Autodesk Fusion 360 part; units mm, degrees
(part 2 of 4)
sketch "Esboço4" plane through (0, 0, 2) normal (0, 0, 1) x (-1, 0, 0)
  arc A0 (-38.7303, -7.6383) -> (-38.142, -9.266) centre (-36.7404, -7.8393) ccw
  arc A1 (-38.7303, -7.6383) -> (-38.7376, 7.7103) centre (-114.3455, 0) ccw
  arc A2 (-38.1438, 9.3455) -> (-38.7376, 7.7103) centre (-36.7479, 7.9132) ccw
  line L0 (-38.1438, 9.3455) -> (-27.9241, 19.3052)
  arc A3 (-24.5283, 17.871) -> (-27.9241, 19.3052) centre (-26.5283, 17.8728) ccw
  line L1 (-24.5283, 17.871) -> (-24.5606, -17.8415)
  arc A4 (-27.9622, -19.2664) -> (-24.5607, -17.8415) centre (-26.5606, -17.8397) ccw
  line L2 (-27.9622, -19.2664) -> (-38.142, -9.266)
  line L3 (19.3052, -27.9241) -> (9.3455, -38.1438)
  arc A5 (7.7103, -38.7376) -> (9.3455, -38.1438) centre (7.9132, -36.7479) ccw
  arc A6 (7.7103, -38.7376) -> (-7.6383, -38.7303) centre (0, -114.3455) ccw
  arc A7 (-9.266, -38.142) -> (-7.6383, -38.7303) centre (-7.8393, -36.7404) ccw
  line L4 (-9.266, -38.142) -> (-19.2664, -27.9622)
  arc A8 (-17.8415, -24.5606) -> (-19.2664, -27.9622) centre (-17.8397, -26.5606) ccw
  line L5 (-17.8415, -24.5606) -> (17.871, -24.5283)
  arc A9 (19.3052, -27.9241) -> (17.871, -24.5283) centre (17.8728, -26.5283) ccw
  arc A10 (37.4337, 15.5639) -> (40.6601, 16.1647) centre (38.8376, 16.9884) ccw
  line L6 (37.4337, 15.5639) -> (14.6425, 38.0264)
  arc A11 (15.1963, 41.2612) -> (14.6425, 38.0264) centre (16.0464, 39.4508) ccw
  line L7 (15.1963, 41.2612) -> (28.3187, 47.4234)
  arc A12 (34.7856, 45.3775) -> (28.3187, 47.4234) centre (30.444, 42.8975) ccw
  arc A13 (34.7856, 45.3775) -> (44.4886, 35.8486) centre (56.4937, 57.7776) ccw
  arc A14 (46.6438, 29.4035) -> (44.4886, 35.8486) centre (42.0875, 31.4628) ccw
  line L8 (46.6438, 29.4035) -> (40.6601, 16.1647)
  line L9 (41.7895, -17.0192) -> (61.9965, -63.6935)
  arc A15 (55.3948, -68.0303) -> (61.9965, -63.6935) centre (58.3475, -65.3318) ccw
  line L10 (55.3948, -68.0303) -> (23.5953, -33.2362)
  arc A16 (23.7067, -29.0729) -> (23.5953, -33.2362) centre (25.8097, -31.2123) ccw
  line L11 (23.7067, -29.0729) -> (36.9334, -16.0716)
  arc A17 (41.7895, -17.0192) -> (36.9334, -16.0716) centre (39.0364, -18.2111) ccw
  arc A18 (9.266, 38.142) -> (7.6383, 38.7303) centre (7.8393, 36.7404) ccw
  line L12 (9.266, 38.142) -> (19.2664, 27.9622)
  arc A19 (17.8415, 24.5606) -> (19.2664, 27.9622) centre (17.8397, 26.5606) ccw
  line L13 (17.8415, 24.5606) -> (-17.871, 24.5283)
  arc A20 (-19.3052, 27.9241) -> (-17.871, 24.5283) centre (-17.8728, 26.5283) ccw
  line L14 (-19.3052, 27.9241) -> (-9.3455, 38.1438)
  arc A21 (-7.7103, 38.7376) -> (-9.3455, 38.1438) centre (-7.9132, 36.7479) ccw
  arc A22 (-7.7103, 38.7376) -> (7.6383, 38.7303) centre (0, 114.3455) ccw
  arc A23 (38.1376, -9.2791) -> (38.7256, -7.6527) centre (36.7356, -7.8528) ccw
  line L15 (38.1376, -9.2791) -> (27.9736, -19.2699)
  arc A24 (24.5716, -17.8424) -> (27.9736, -19.2699) centre (26.5716, -17.8436) ccw
  line L16 (24.5716, -17.8424) -> (24.5916, 17.8264)
  arc A25 (27.9955, 19.2498) -> (24.5916, 17.8264) centre (26.5916, 17.8253) ccw
  line L17 (27.9955, 19.2498) -> (38.1463, 9.2454)
  arc A26 (38.7321, 7.6192) -> (38.1463, 9.2454) centre (36.7424, 7.821) ccw
  arc A27 (38.7321, 7.6192) -> (38.7256, -7.6527) centre (114.3432, -0.0492) ccw
  arc A28 (-61.9967, -63.6938) -> (-55.4143, -68.0759) centre (-58.3695, -65.3802) ccw
  line L18 (-61.9967, -63.6938) -> (-41.8922, -17.2564)
  arc A29 (-36.246, -16.5772) -> (-41.8922, -17.2564) centre (-38.8636, -18.6251) ccw
  line L19 (-36.246, -16.5772) -> (-23.6374, -29.1331)
  arc A30 (-23.5625, -33.2372) -> (-23.6374, -29.1331) centre (-25.7596, -31.2246) ccw
  line L20 (-23.5625, -33.2372) -> (-55.4143, -68.0759)
  line L21 (5, -97.464) -> (5, -58.6595)
  arc A31 (7, -56.6595) -> (5, -58.6595) centre (7, -58.6595) ccw
  line L22 (7, -56.6595) -> (10.473, -56.6595)
  arc A32 (14.3032, -58.4456) -> (10.473, -56.6595) centre (10.473, -61.6595) ccw
  line L23 (14.3032, -58.4456) -> (34.3305, -82.3132)
  arc A33 (35.4243, -86.3954) -> (34.3305, -82.3132) centre (30.5003, -85.5271) ccw
  line L24 (35.4243, -86.3954) -> (32.7648, -101.4781)
  arc A34 (26.9725, -105.5339) -> (32.7648, -101.4781) centre (27.8408, -100.6098) ccw
  line L25 (26.9725, -105.5339) -> (9.1318, -102.3881)
  arc A35 (5, -97.464) -> (9.1318, -102.3881) centre (10, -97.464) ccw
  arc A36 (-40.9054, 16.7074) -> (-37.3489, 15.6517) centre (-38.8619, 17.0732) ccw
  line L26 (-40.9054, 16.7074) -> (-46.7322, 29.5993)
  arc A37 (-44.339, 36.0244) -> (-46.7322, 29.5993) centre (-42.0339, 31.5075) ccw
  arc A38 (-44.339, 36.0244) -> (-34.6129, 45.4956) centre (-56.2565, 57.9923) ccw
  arc A39 (-28.1234, 47.5076) -> (-34.6129, 45.4956) centre (-30.28, 42.9921) ccw
  line L27 (-28.1234, 47.5076) -> (-14.9942, 41.2515)
  arc A40 (-14.46, 38.0146) -> (-14.9942, 41.2515) centre (-15.8549, 39.4469) ccw
  line L28 (-14.46, 38.0146) -> (-37.3489, 15.6517)
  line L29 (70.4711, -73.2) -> (50.5773, -27.2494)
  arc A41 (51.0282, 29.3922) -> (50.5773, -27.2494) centre (114.8154, 0.5617) ccw
  line L30 (51.0282, 29.3922) -> (70.7852, 73.1043)
  arc A42 (70.7852, 73.1043) -> (60.1979, 89.9288) centre (75, 87.5) ccw
  arc A43 (35.9657, 79.8952) -> (60.1979, 89.9288) centre (-0.31, 201.7835) ccw
  arc A44 (-60.2098, 89.9999) -> (-70.7852, 73.1043) centre (-75, 87.5) ccw
  line L31 (-70.7852, 73.1043) -> (-51.0282, 29.3922)
  arc A45 (-50.5773, -27.2494) -> (-51.0282, 29.3922) centre (-114.8154, 0.5617) ccw
  line L32 (-50.5773, -27.2494) -> (-70.4711, -73.2)
  arc A46 (-70.4711, -73.2) -> (-73.7447, -102.4474) centre (-75, -87.5) ccw
  arc A47 (-46.7294, -108.889) -> (-73.7447, -102.4474) centre (-70.0264, -146.7235) ccw
  arc A48 (72.6915, -102.3213) -> (44.7852, -108.3244) centre (66.5604, -141.6847) ccw
  arc A49 (72.6915, -102.3213) -> (70.4711, -73.2) centre (75, -87.5) ccw
  arc A50 (-10.473, -56.6595) -> (-14.3032, -58.4456) centre (-10.473, -61.6595) ccw
  line L33 (-10.473, -56.6595) -> (-7, -56.6595)
  arc A51 (-5, -58.6595) -> (-7, -56.6595) centre (-7, -58.6595) ccw
  line L34 (-5, -58.6595) -> (-5, -97.464)
  arc A52 (-9.1318, -102.3881) -> (-5, -97.464) centre (-10, -97.464) ccw
  line L35 (-9.1318, -102.3881) -> (-26.9725, -105.5339)
  arc A53 (-32.7648, -101.4781) -> (-26.9725, -105.5339) centre (-27.8408, -100.6098) ccw
  line L36 (-32.7648, -101.4781) -> (-35.4243, -86.3954)
  arc A54 (-34.3305, -82.3132) -> (-35.4243, -86.3954) centre (-30.5003, -85.5271) ccw
  line L37 (-34.3305, -82.3132) -> (-14.3032, -58.4456)
  circle A55 centre (-40.65, 60) radius 2.15
  line L38 (47.15, 42.4858) -> (47.15, 67.561)
  arc A56 (49.4611, 71.7764) -> (47.15, 67.561) centre (52.15, 67.561) ccw
  line L39 (49.4611, 71.7764) -> (57.5607, 76.943)
  arc A57 (64.8173, 70.6939) -> (57.5607, 76.943) centre (60.2496, 72.7276) ccw
  line L40 (64.8173, 70.6939) -> (51.1653, 40.0309)
  arc A58 (49.5538, 39.7214) -> (51.1653, 40.0309) centre (50.2517, 40.4376) ccw
  line L41 (49.5538, 39.7214) -> (47.4521, 41.7697)
  arc A59 (47.15, 42.4858) -> (47.4521, 41.7697) centre (48.15, 42.4858) ccw
  circle A60 centre (40.65, 60) radius 2.15
  circle A61 centre (-40.65, 50) radius 2.15
  arc A62 (-57.5607, 76.943) -> (-64.8173, 70.6939) centre (-60.2496, 72.7276) ccw
  line L42 (-57.5607, 76.943) -> (-49.4611, 71.7764)
  arc A63 (-47.15, 67.561) -> (-49.4611, 71.7764) centre (-52.15, 67.561) ccw
  line L43 (-47.15, 67.561) -> (-47.15, 42.4858)
  arc A64 (-47.4521, 41.7697) -> (-47.15, 42.4858) centre (-48.15, 42.4858) ccw
  line L44 (-47.4521, 41.7697) -> (-49.5538, 39.7214)
  arc A65 (-51.1653, 40.0309) -> (-49.5538, 39.7214) centre (-50.2517, 40.4376) ccw
  line L45 (-51.1653, 40.0309) -> (-64.8173, 70.6939)
  circle A66 centre (40.65, 50) radius 2.15
  line L46 (8, -50.7) -> (-8, -42.5) construction
  line L47 (0, -46.6) -> (-20, -46.6) construction
  arc A67 (-9.266, -38.142) -> (-7.6383, -38.7303) centre (-7.8393, -36.7404) ccw
  line L48 (-8, -50.7) -> (-8, -42.5)
  line L49 (-8, -42.5) -> (8, -42.5)
  circle A68 centre (-10.25, -46.6) radius 1.5
  line L50 (8, -50.7) -> (-8, -50.7)
  line L51 (0, -46.6) -> (20, -46.6) construction
  arc A69 (7.7103, -38.7376) -> (9.3455, -38.1438) centre (7.9132, -36.7479) ccw
  line L52 (-8, -50.7) -> (8, -42.5) construction
  arc A70 (7.7103, -38.7376) -> (-7.6383, -38.7303) centre (0, -114.3455) ccw
  line L53 (8, -42.5) -> (8, -50.7)
  circle A71 centre (10.25, -46.6) radius 1.5
  line L54 (8.1464, -6.7322) -> (2.1213, -0.7071)
  arc A72 (2.1213, 0.7071) -> (2.1213, -0.7071) centre (2.8284, 0) ccw
  line L55 (2.1213, 0.7071) -> (8.1464, 6.7322)
  arc A73 (9, 6.3787) -> (8.1464, 6.7322) centre (8.5, 6.3787) ccw
  line L56 (9, 6.3787) -> (9, -6.3787)
  arc A74 (8.1464, -6.7322) -> (9, -6.3787) centre (8.5, -6.3787) ccw
  arc A75 (-6.7322, -8.1464) -> (-6.3787, -9) centre (-6.3787, -8.5) ccw
  line L57 (-6.7322, -8.1464) -> (-0.7071, -2.1213)
  arc A76 (0.7071, -2.1213) -> (-0.7071, -2.1213) centre (0, -2.8284) ccw
  line L58 (0.7071, -2.1213) -> (6.7322, -8.1464)
  arc A77 (6.3787, -9) -> (6.7322, -8.1464) centre (6.3787, -8.5) ccw
  line L59 (6.3787, -9) -> (-6.3787, -9)
  arc A78 (-8.1464, 6.7322) -> (-9, 6.3787) centre (-8.5, 6.3787) ccw
  line L60 (-8.1464, 6.7322) -> (-2.1213, 0.7071)
  arc A79 (-2.1213, -0.7071) -> (-2.1213, 0.7071) centre (-2.8284, 0) ccw
  line L61 (-2.1213, -0.7071) -> (-8.1464, -6.7322)
  arc A80 (-9, -6.3787) -> (-8.1464, -6.7322) centre (-8.5, -6.3787) ccw
  line L62 (-9, -6.3787) -> (-9, 6.3787)
  arc A81 (6.7322, 8.1464) -> (6.3787, 9) centre (6.3787, 8.5) ccw
  line L63 (6.7322, 8.1464) -> (0.7071, 2.1213)
  arc A82 (-0.7071, 2.1213) -> (0.7071, 2.1213) centre (0, 2.8284) ccw
  line L64 (-0.7071, 2.1213) -> (-6.7322, 8.1464)
  arc A83 (-6.3787, 9) -> (-6.7322, 8.1464) centre (-6.3787, 8.5) ccw
  line L65 (-6.3787, 9) -> (6.3787, 9)
  line L66 (35.9657, 79.8952) -> (2.1827, 93.0889)
  arc A84 (2.1827, 93.0889) -> (-2.1423, 93.1045) centre (0, 87.5) ccw
  line L67 (0, 81.5) -> (15.6612, 75.3836)
  line L68 (-16.4256, 75.2214) -> (0, 81.5)
  line L69 (-2.1423, 93.1045) -> (-36.9275, 79.8081)
  arc A85 (-60.2098, 89.9999) -> (-36.7745, 80.3179) centre (-0.31, 201.7835) ccw
  circle A86 centre (0, 87.5) radius 2.15
  arc A87 (26.2105, 50.915) -> (27.5676, 55.0697) centre (24.9353, 53.6305) ccw
  line L70 (26.2105, 50.915) -> (10.6059, 43.5872)
  arc A88 (9.3307, 43.3027) -> (10.6059, 43.5872) centre (9.3307, 46.3027) ccw
  line L71 (9.3307, 43.3027) -> (-9.3218, 43.3027)
  arc A89 (-10.6123, 43.5944) -> (-9.3218, 43.3027) centre (-9.3218, 46.3027) ccw
  line L72 (-10.6123, 43.5944) -> (-26.8632, 51.3381)
  arc A90 (-28.1945, 55.5044) -> (-26.8632, 51.3381) centre (-25.5727, 54.0463) ccw
  line L73 (-28.1945, 55.5044) -> (-17.9762, 73.8773)
  arc A91 (-16.4256, 75.2214) -> (-17.9762, 73.8773) centre (-15.3544, 72.4192) ccw
  arc A92 (17.2021, 74.0283) -> (15.6612, 75.3836) centre (14.5698, 72.5892) ccw
  line L74 (17.2021, 74.0283) -> (27.5676, 55.0697)
  arc A93 (-46.7294, -108.889) -> (-25.7561, -114.8285) centre (-25.7561, -74.8285) ccw
  line L75 (-25.7561, -114.8285) -> (22.9214, -114.8285)
  arc A94 (22.9214, -114.8285) -> (44.7852, -108.3244) centre (22.9214, -74.8285) ccw
  circle A95 centre (10, 10) radius 3
  circle A96 centre (-10, -10) radius 3
  circle A97 centre (10, -10) radius 3
  circle A98 centre (-10, 10) radius 3
  point P0 (0, -46.6)
  point P1 (0.156, 201.9423)
  point P2 (0.156, 201.9423)
  point P3 (0.156, 201.9423)
  point P4 (0.2929, 201.9885)
  point P5 (0.2929, 201.9885)
  point P6 (0.2929, 201.9885)
  point P7 (2.2046, 200.8918)
  point P8 (2.2046, 200.8918)
  dimension "d91" = 16
  dimension "d92" = 8.2
  dimension "d93" = 3
  dimension "d94" = 2.25
  dimension "d96" = 42.5
  dimension "d97" = 2.25
  constraint horizontal L50
  constraint perpendicular L48 L50
  constraint parallel L49 L50
  constraint parallel L48 L53
  constraint coincident P0 L46
  constraint coincident P0 L52
  constraint coincident P0 L47.start
  constraint perpendicular L47 L48
  constraint perpendicular L51 L53
  constraint coincident A71.centre L51
  measures "d91" distance of L46.end L49.end
  measures "d92" distance of L46.end L48.start
  measures "d93" diameter of A71
  measures "d94" distance of A71.centre L53
  measures "d96" distance of origin L49
  measures "d97" distance of A68.centre L48
extrude "Extrusão4" cut sketch "Esboço4" against normal through all contours L48 L49 L50 L53 | A68 | A71
sketch "Esboço5" plane through (0, 0, 2) normal (0, 0, 1) x (-1, 0, 0)
  circle A0 centre (40.65, 50) radius 2.15
  arc A1 (-57.5607, 76.943) -> (-64.8173, 70.6939) centre (-60.2496, 72.7276) ccw
  line L0 (-57.5607, 76.943) -> (-49.4611, 71.7764)
  arc A2 (-47.15, 67.561) -> (-49.4611, 71.7764) centre (-52.15, 67.561) ccw
  line L1 (-47.15, 67.561) -> (-47.15, 42.4858)
  arc A3 (-47.4521, 41.7697) -> (-47.15, 42.4858) centre (-48.15, 42.4858) ccw
  line L2 (-47.4521, 41.7697) -> (-49.5538, 39.7214)
  arc A4 (-51.1653, 40.0309) -> (-49.5538, 39.7214) centre (-50.2517, 40.4376) ccw
  line L3 (-51.1653, 40.0309) -> (-64.8173, 70.6939)
  circle A5 centre (-40.65, 50) radius 2.15
  circle A6 centre (40.65, 60) radius 2.15
  line L4 (47.15, 42.4858) -> (47.15, 67.561)
  arc A7 (49.4611, 71.7764) -> (47.15, 67.561) centre (52.15, 67.561) ccw
  line L5 (49.4611, 71.7764) -> (57.5607, 76.943)
  arc A8 (64.8173, 70.6939) -> (57.5607, 76.943) centre (60.2496, 72.7276) ccw
  line L6 (64.8173, 70.6939) -> (51.1653, 40.0309)
  arc A9 (49.5538, 39.7214) -> (51.1653, 40.0309) centre (50.2517, 40.4376) ccw
  line L7 (49.5538, 39.7214) -> (47.4521, 41.7697)
  arc A10 (47.15, 42.4858) -> (47.4521, 41.7697) centre (48.15, 42.4858) ccw
  circle A11 centre (-40.65, 60) radius 2.15
  arc A12 (-10.473, -56.6595) -> (-14.3032, -58.4456) centre (-10.473, -61.6595) ccw
  line L8 (-10.473, -56.6595) -> (-7, -56.6595)
  arc A13 (-5, -58.6595) -> (-7, -56.6595) centre (-7, -58.6595) ccw
  line L9 (-5, -58.6595) -> (-5, -97.464)
  arc A14 (-9.1318, -102.3881) -> (-5, -97.464) centre (-10, -97.464) ccw
  line L10 (-9.1318, -102.3881) -> (-26.9725, -105.5339)
  arc A15 (-32.7648, -101.4781) -> (-26.9725, -105.5339) centre (-27.8408, -100.6098) ccw
  line L11 (-32.7648, -101.4781) -> (-35.4243, -86.3954)
  arc A16 (-34.3305, -82.3132) -> (-35.4243, -86.3954) centre (-30.5003, -85.5271) ccw
  line L12 (-34.3305, -82.3132) -> (-14.3032, -58.4456)
  line L13 (70.4711, -73.2) -> (50.5773, -27.2494)
  arc A17 (51.0282, 29.3922) -> (50.5773, -27.2494) centre (114.8154, 0.5617) ccw
  line L14 (51.0282, 29.3922) -> (70.7852, 73.1043)
  arc A18 (70.7852, 73.1043) -> (60.1979, 89.9288) centre (75, 87.5) ccw
  arc A19 (35.9657, 79.8952) -> (60.1979, 89.9288) centre (-0.31, 201.7835) ccw
  arc A20 (-60.2098, 89.9999) -> (-70.7852, 73.1043) centre (-75, 87.5) ccw
  line L15 (-70.7852, 73.1043) -> (-51.0282, 29.3922)
  arc A21 (-50.5773, -27.2494) -> (-51.0282, 29.3922) centre (-114.8154, 0.5617) ccw
  line L16 (-50.5773, -27.2494) -> (-70.4711, -73.2)
  arc A22 (-70.4711, -73.2) -> (-73.7447, -102.4474) centre (-75, -87.5) ccw
  arc A23 (-46.7294, -108.889) -> (-73.7447, -102.4474) centre (-70.0264, -146.7235) ccw
  arc A24 (72.6915, -102.3213) -> (44.7852, -108.3244) centre (66.5604, -141.6847) ccw
  arc A25 (72.6915, -102.3213) -> (70.4711, -73.2) centre (75, -87.5) ccw
  arc A26 (-40.9054, 16.7074) -> (-37.3489, 15.6517) centre (-38.8619, 17.0732) ccw
  line L17 (-40.9054, 16.7074) -> (-46.7322, 29.5993)
  arc A27 (-44.339, 36.0244) -> (-46.7322, 29.5993) centre (-42.0339, 31.5075) ccw
  arc A28 (-44.339, 36.0244) -> (-34.6129, 45.4956) centre (-56.2565, 57.9923) ccw
  arc A29 (-28.1234, 47.5076) -> (-34.6129, 45.4956) centre (-30.28, 42.9921) ccw
  line L18 (-28.1234, 47.5076) -> (-14.9942, 41.2515)
  arc A30 (-14.46, 38.0146) -> (-14.9942, 41.2515) centre (-15.8549, 39.4469) ccw
  line L19 (-14.46, 38.0146) -> (-37.3489, 15.6517)
  line L20 (5, -97.464) -> (5, -58.6595)
  arc A31 (7, -56.6595) -> (5, -58.6595) centre (7, -58.6595) ccw
  line L21 (7, -56.6595) -> (10.473, -56.6595)
  arc A32 (14.3032, -58.4456) -> (10.473, -56.6595) centre (10.473, -61.6595) ccw
  line L22 (14.3032, -58.4456) -> (34.3305, -82.3132)
  arc A33 (35.4243, -86.3954) -> (34.3305, -82.3132) centre (30.5003, -85.5271) ccw
  line L23 (35.4243, -86.3954) -> (32.7648, -101.4781)
  arc A34 (26.9725, -105.5339) -> (32.7648, -101.4781) centre (27.8408, -100.6098) ccw
  line L24 (26.9725, -105.5339) -> (9.1318, -102.3881)
  arc A35 (5, -97.464) -> (9.1318, -102.3881) centre (10, -97.464) ccw
  arc A36 (-61.9967, -63.6938) -> (-55.4143, -68.0759) centre (-58.3695, -65.3802) ccw
  line L25 (-61.9967, -63.6938) -> (-41.8922, -17.2564)
  arc A37 (-36.246, -16.5772) -> (-41.8922, -17.2564) centre (-38.8636, -18.6251) ccw
  line L26 (-36.246, -16.5772) -> (-23.6374, -29.1331)
  arc A38 (-23.5625, -33.2372) -> (-23.6374, -29.1331) centre (-25.7596, -31.2246) ccw
  line L27 (-23.5625, -33.2372) -> (-55.4143, -68.0759)
  arc A39 (38.1376, -9.2791) -> (38.7256, -7.6527) centre (36.7356, -7.8528) ccw
  line L28 (38.1376, -9.2791) -> (27.9736, -19.2699)
  arc A40 (24.5716, -17.8424) -> (27.9736, -19.2699) centre (26.5716, -17.8436) ccw
  line L29 (24.5716, -17.8424) -> (24.5916, 17.8264)
  arc A41 (27.9955, 19.2498) -> (24.5916, 17.8264) centre (26.5916, 17.8253) ccw
  line L30 (27.9955, 19.2498) -> (38.1463, 9.2454)
  arc A42 (38.7321, 7.6192) -> (38.1463, 9.2454) centre (36.7424, 7.821) ccw
  arc A43 (38.7321, 7.6192) -> (38.7256, -7.6527) centre (114.3432, -0.0492) ccw
  arc A44 (9.266, 38.142) -> (7.6383, 38.7303) centre (7.8393, 36.7404) ccw
  line L31 (9.266, 38.142) -> (19.2664, 27.9622)
  arc A45 (17.8415, 24.5606) -> (19.2664, 27.9622) centre (17.8397, 26.5606) ccw
  line L32 (17.8415, 24.5606) -> (-17.871, 24.5283)
  arc A46 (-19.3052, 27.9241) -> (-17.871, 24.5283) centre (-17.8728, 26.5283) ccw
  line L33 (-19.3052, 27.9241) -> (-9.3455, 38.1438)
  arc A47 (-7.7103, 38.7376) -> (-9.3455, 38.1438) centre (-7.9132, 36.7479) ccw
  arc A48 (-7.7103, 38.7376) -> (7.6383, 38.7303) centre (0, 114.3455) ccw
  line L34 (41.7895, -17.0192) -> (61.9965, -63.6935)
  arc A49 (55.3948, -68.0303) -> (61.9965, -63.6935) centre (58.3475, -65.3318) ccw
  line L35 (55.3948, -68.0303) -> (23.5953, -33.2362)
  arc A50 (23.7067, -29.0729) -> (23.5953, -33.2362) centre (25.8097, -31.2123) ccw
  line L36 (23.7067, -29.0729) -> (36.9334, -16.0716)
  arc A51 (41.7895, -17.0192) -> (36.9334, -16.0716) centre (39.0364, -18.2111) ccw
  arc A52 (37.4337, 15.5639) -> (40.6601, 16.1647) centre (38.8376, 16.9884) ccw
  line L37 (37.4337, 15.5639) -> (14.6425, 38.0264)
  arc A53 (15.1963, 41.2612) -> (14.6425, 38.0264) centre (16.0464, 39.4508) ccw
  line L38 (15.1963, 41.2612) -> (28.3187, 47.4234)
  arc A54 (34.7856, 45.3775) -> (28.3187, 47.4234) centre (30.444, 42.8975) ccw
  arc A55 (34.7856, 45.3775) -> (44.4886, 35.8486) centre (56.4937, 57.7776) ccw
  arc A56 (46.6438, 29.4035) -> (44.4886, 35.8486) centre (42.0875, 31.4628) ccw
  line L39 (46.6438, 29.4035) -> (40.6601, 16.1647)
  line L40 (19.3052, -27.9241) -> (9.3455, -38.1438)
  arc A57 (7.7103, -38.7376) -> (9.3455, -38.1438) centre (7.9132, -36.7479) ccw
  arc A58 (7.7103, -38.7376) -> (-7.6383, -38.7303) centre (0, -114.3455) ccw
  arc A59 (-9.266, -38.142) -> (-7.6383, -38.7303) centre (-7.8393, -36.7404) ccw
  line L41 (-9.266, -38.142) -> (-19.2664, -27.9622)
  arc A60 (-17.8415, -24.5606) -> (-19.2664, -27.9622) centre (-17.8397, -26.5606) ccw
  line L42 (-17.8415, -24.5606) -> (17.871, -24.5283)
  arc A61 (19.3052, -27.9241) -> (17.871, -24.5283) centre (17.8728, -26.5283) ccw
  arc A62 (-38.7303, -7.6383) -> (-38.142, -9.266) centre (-36.7404, -7.8393) ccw
  arc A63 (-38.7303, -7.6383) -> (-38.7376, 7.7103) centre (-114.3455, 0) ccw
  arc A64 (-38.1438, 9.3455) -> (-38.7376, 7.7103) centre (-36.7479, 7.9132) ccw
  line L43 (-38.1438, 9.3455) -> (-27.9241, 19.3052)
  arc A65 (-24.5283, 17.871) -> (-27.9241, 19.3052) centre (-26.5283, 17.8728) ccw
  line L44 (-24.5283, 17.871) -> (-24.5606, -17.8415)
  arc A66 (-27.9622, -19.2664) -> (-24.5607, -17.8415) centre (-26.5606, -17.8397) ccw
  line L45 (-27.9622, -19.2664) -> (-38.142, -9.266)
  circle A67 centre (-10.25, -46.6) radius 1.5
  line L46 (8, -42.5) -> (8, -50.7)
  line L47 (8, -50.7) -> (-8, -50.7)
  line L48 (-8, -50.7) -> (-8, -42.5)
  line L49 (-8, -42.5) -> (8, -42.5)
  circle A68 centre (10.25, -46.6) radius 1.5
  circle A69 centre (75, 87.5) radius 3
  circle A70 centre (-75, 87.5) radius 3
  circle A71 centre (72.5, -87.6021) radius 3
  circle A72 centre (-75, -87.5) radius 3
  circle A73 centre (72.5, -95.6021) radius 1.5
  circle A74 centre (80.5, -87.6021) radius 1.5
  circle A75 centre (72.5, -79.6021) radius 1.5
  circle A76 centre (64.5, -87.6021) radius 1.5
  circle A77 centre (-74.9995, -95.5) radius 1.5
  circle A78 centre (-67, -87.4995) radius 1.5
  circle A79 centre (-75.0005, -79.5) radius 1.5
  circle A80 centre (-83, -87.5005) radius 1.5
  circle A81 centre (75, 95.5) radius 1.5
  circle A82 centre (67, 87.5) radius 1.5
  circle A83 centre (75, 79.5) radius 1.5
  circle A84 centre (83, 87.5) radius 1.5
  circle A85 centre (-75.0002, 95.5) radius 1.5
  circle A86 centre (-83, 87.4998) radius 1.5
  circle A87 centre (-74.9998, 79.5) radius 1.5
  circle A88 centre (-67, 87.5002) radius 1.5
  line L50 (35.9657, 79.8952) -> (2.1827, 93.0889)
  arc A89 (2.1827, 93.0889) -> (-2.1423, 93.1045) centre (0, 87.5) ccw
  line L51 (0, 81.5) -> (15.6612, 75.3836)
  line L52 (-16.4256, 75.2214) -> (0, 81.5)
  line L53 (-2.1423, 93.1045) -> (-36.9275, 79.8081)
  arc A90 (-60.2098, 89.9999) -> (-36.7745, 80.3179) centre (-0.31, 201.7835) ccw
  arc A91 (6.7322, 8.1464) -> (6.3787, 9) centre (6.3787, 8.5) ccw
  line L54 (6.7322, 8.1464) -> (0.7071, 2.1213)
  arc A92 (-0.7071, 2.1213) -> (0.7071, 2.1213) centre (0, 2.8284) ccw
  line L55 (-0.7071, 2.1213) -> (-6.7322, 8.1464)
  arc A93 (-6.3787, 9) -> (-6.7322, 8.1464) centre (-6.3787, 8.5) ccw
  line L56 (-6.3787, 9) -> (6.3787, 9)
  arc A94 (-8.1464, 6.7322) -> (-9, 6.3787) centre (-8.5, 6.3787) ccw
  line L57 (-8.1464, 6.7322) -> (-2.1213, 0.7071)
  arc A95 (-2.1213, -0.7071) -> (-2.1213, 0.7071) centre (-2.8284, 0) ccw
  line L58 (-2.1213, -0.7071) -> (-8.1464, -6.7322)
  arc A96 (-9, -6.3787) -> (-8.1464, -6.7322) centre (-8.5, -6.3787) ccw
  line L59 (-9, -6.3787) -> (-9, 6.3787)
  arc A97 (-6.7322, -8.1464) -> (-6.3787, -9) centre (-6.3787, -8.5) ccw
  line L60 (-6.7322, -8.1464) -> (-0.7071, -2.1213)
  arc A98 (0.7071, -2.1213) -> (-0.7071, -2.1213) centre (0, -2.8284) ccw
  line L61 (0.7071, -2.1213) -> (6.7322, -8.1464)
  arc A99 (6.3787, -9) -> (6.7322, -8.1464) centre (6.3787, -8.5) ccw
  line L62 (6.3787, -9) -> (-6.3787, -9)
  line L63 (8.1464, -6.7322) -> (2.1213, -0.7071)
  arc A100 (2.1213, 0.7071) -> (2.1213, -0.7071) centre (2.8284, 0) ccw
  line L64 (2.1213, 0.7071) -> (8.1464, 6.7322)
  arc A101 (9, 6.3787) -> (8.1464, 6.7322) centre (8.5, 6.3787) ccw
  line L65 (9, 6.3787) -> (9, -6.3787)
  arc A102 (8.1464, -6.7322) -> (9, -6.3787) centre (8.5, -6.3787) ccw
  circle A103 centre (0, 87.5) radius 2.15
  arc A104 (26.2105, 50.915) -> (27.5676, 55.0697) centre (24.9353, 53.6305) ccw
  line L66 (26.2105, 50.915) -> (10.6059, 43.5872)
  arc A105 (9.3307, 43.3027) -> (10.6059, 43.5872) centre (9.3307, 46.3027) ccw
  line L67 (9.3307, 43.3027) -> (-9.3218, 43.3027)
  arc A106 (-10.6123, 43.5944) -> (-9.3218, 43.3027) centre (-9.3218, 46.3027) ccw
  line L68 (-10.6123, 43.5944) -> (-26.8632, 51.3381)
  arc A107 (-28.1945, 55.5044) -> (-26.8632, 51.3381) centre (-25.5727, 54.0463) ccw
  line L69 (-28.1945, 55.5044) -> (-17.9762, 73.8773)
  arc A108 (-16.4256, 75.2214) -> (-17.9762, 73.8773) centre (-15.3544, 72.4192) ccw
  arc A109 (17.2021, 74.0283) -> (15.6612, 75.3836) centre (14.5698, 72.5892) ccw
  line L70 (17.2021, 74.0283) -> (27.5676, 55.0697)
  arc A110 (-46.7294, -108.889) -> (-25.7561, -114.8285) centre (-25.7561, -74.8285) ccw
  line L71 (-25.7561, -114.8285) -> (22.9214, -114.8285)
  arc A111 (22.9214, -114.8285) -> (44.7852, -108.3244) centre (22.9214, -74.8285) ccw
  circle A112 centre (-10, 10) radius 3
  circle A113 centre (10, -10) radius 3
  circle A114 centre (-10, -10) radius 3
  circle A115 centre (10, 10) radius 3
  circle A116 centre (-75, -87.5) radius 15
  circle A117 centre (75, 87.5) radius 15
  point P0 (0.156, 201.9423)
  point P1 (0.156, 201.9423)
  point P2 (0.156, 201.9423)
  point P3 (0.2929, 201.9885)
  point P4 (0.2929, 201.9885)
  point P5 (0.2929, 201.9885)
  point P6 (2.2046, 200.8918)
  point P7 (2.2046, 200.8918)
  dimension "d99" = 6
  dimension "d100" = 6
  dimension "d101" = 6
  dimension "d102" = 6
  dimension "d103" = 3
  dimension "d104" = 8
  dimension "d106" = 360
  dimension "d107" = 3
  dimension "d108" = 8
  dimension "d110" = 360
  dimension "d111" = 3
  dimension "d112" = 8
  dimension "d114" = 360
  dimension "d115" = 3
  dimension "d116" = 8
  dimension "d118" = 360
  constraint concentric A20 A70
  constraint concentric A72 A116
  constraint concentric A69 A117
  measures "d99" diameter of A69
  measures "d100" diameter of A70
  measures "d101" diameter of A71
  measures "d102" diameter of A72
  measures "d103" diameter of A73
  measures "d104" distance of A71.centre A73.centre
  measures "d107" diameter of A77
  measures "d108" distance of A22.centre A77.centre
  measures "d111" diameter of A81
  measures "d112" distance of A18.centre A81.centre
  measures "d115" diameter of A85
  measures "d116" distance of A20.centre A85.centre
extrude "Extrusão5" cut sketch "Esboço5" against normal through all contours A69 | A70 | A71 | A72 | A73 | A74 | A75 | A76 | A77 | A78 | A79 | A80 | A81 | A82 | A83 | A84 | A85 | A86 | A87 | A88
sketch "Esboço6" plane through (0, 0, 2) normal (0, 0, 1) x (-1, 0, 0)
  circle A0 centre (10.25, -46.6) radius 1.5
  line L0 (8, -42.5) -> (8, -50.7)
  line L1 (8, -50.7) -> (-8, -50.7)
  line L2 (-8, -50.7) -> (-8, -42.5)
  line L3 (-8, -42.5) -> (8, -42.5)
  circle A1 centre (-10.25, -46.6) radius 1.5
  arc A2 (-38.7303, -7.6383) -> (-38.142, -9.266) centre (-36.7404, -7.8393) ccw
  arc A3 (-38.7303, -7.6383) -> (-38.7376, 7.7103) centre (-114.3455, 0) ccw
  arc A4 (-38.1438, 9.3455) -> (-38.7376, 7.7103) centre (-36.7479, 7.9132) ccw
  line L4 (-38.1438, 9.3455) -> (-27.9241, 19.3052)
  arc A5 (-24.5283, 17.871) -> (-27.9241, 19.3052) centre (-26.5283, 17.8728) ccw
  line L5 (-24.5283, 17.871) -> (-24.5606, -17.8415)
  arc A6 (-27.9622, -19.2664) -> (-24.5607, -17.8415) centre (-26.5606, -17.8397) ccw
  line L6 (-27.9622, -19.2664) -> (-38.142, -9.266)
  line L7 (19.3052, -27.9241) -> (9.3455, -38.1438)
  arc A7 (7.7103, -38.7376) -> (9.3455, -38.1438) centre (7.9132, -36.7479) ccw
  arc A8 (7.7103, -38.7376) -> (-7.6383, -38.7303) centre (0, -114.3455) ccw
  arc A9 (-9.266, -38.142) -> (-7.6383, -38.7303) centre (-7.8393, -36.7404) ccw
  line L8 (-9.266, -38.142) -> (-19.2664, -27.9622)
  arc A10 (-17.8415, -24.5606) -> (-19.2664, -27.9622) centre (-17.8397, -26.5606) ccw
  line L9 (-17.8415, -24.5606) -> (17.871, -24.5283)
  arc A11 (19.3052, -27.9241) -> (17.871, -24.5283) centre (17.8728, -26.5283) ccw
  arc A12 (37.4337, 15.5639) -> (40.6601, 16.1647) centre (38.8376, 16.9884) ccw
  line L10 (37.4337, 15.5639) -> (14.6425, 38.0264)
  arc A13 (15.1963, 41.2612) -> (14.6425, 38.0264) centre (16.0464, 39.4508) ccw
  line L11 (15.1963, 41.2612) -> (28.3187, 47.4234)
  arc A14 (34.7856, 45.3775) -> (28.3187, 47.4234) centre (30.444, 42.8975) ccw
  arc A15 (34.7856, 45.3775) -> (44.4886, 35.8486) centre (56.4937, 57.7776) ccw
  arc A16 (46.6438, 29.4035) -> (44.4886, 35.8486) centre (42.0875, 31.4628) ccw
  line L12 (46.6438, 29.4035) -> (40.6601, 16.1647)
  line L13 (41.7895, -17.0192) -> (61.9965, -63.6935)
  arc A17 (55.3948, -68.0303) -> (61.9965, -63.6935) centre (58.3475, -65.3318) ccw
  line L14 (55.3948, -68.0303) -> (23.5953, -33.2362)
  arc A18 (23.7067, -29.0729) -> (23.5953, -33.2362) centre (25.8097, -31.2123) ccw
  line L15 (23.7067, -29.0729) -> (36.9334, -16.0716)
  arc A19 (41.7895, -17.0192) -> (36.9334, -16.0716) centre (39.0364, -18.2111) ccw
  arc A20 (9.266, 38.142) -> (7.6383, 38.7303) centre (7.8393, 36.7404) ccw
  line L16 (9.266, 38.142) -> (19.2664, 27.9622)
  arc A21 (17.8415, 24.5606) -> (19.2664, 27.9622) centre (17.8397, 26.5606) ccw
  line L17 (17.8415, 24.5606) -> (-17.871, 24.5283)
  arc A22 (-19.3052, 27.9241) -> (-17.871, 24.5283) centre (-17.8728, 26.5283) ccw
  line L18 (-19.3052, 27.9241) -> (-9.3455, 38.1438)
  arc A23 (-7.7103, 38.7376) -> (-9.3455, 38.1438) centre (-7.9132, 36.7479) ccw
  arc A24 (-7.7103, 38.7376) -> (7.6383, 38.7303) centre (0, 114.3455) ccw
  arc A25 (38.1376, -9.2791) -> (38.7256, -7.6527) centre (36.7356, -7.8528) ccw
  line L19 (38.1376, -9.2791) -> (27.9736, -19.2699)
  arc A26 (24.5716, -17.8424) -> (27.9736, -19.2699) centre (26.5716, -17.8436) ccw
  line L20 (24.5716, -17.8424) -> (24.5916, 17.8264)
  arc A27 (27.9955, 19.2498) -> (24.5916, 17.8264) centre (26.5916, 17.8253) ccw
  line L21 (27.9955, 19.2498) -> (38.1463, 9.2454)
  arc A28 (38.7321, 7.6192) -> (38.1463, 9.2454) centre (36.7424, 7.821) ccw
  arc A29 (38.7321, 7.6192) -> (38.7256, -7.6527) centre (114.3432, -0.0492) ccw
  arc A30 (-61.9967, -63.6938) -> (-55.4143, -68.0759) centre (-58.3695, -65.3802) ccw
  line L22 (-61.9967, -63.6938) -> (-41.8922, -17.2564)
  arc A31 (-36.246, -16.5772) -> (-41.8922, -17.2564) centre (-38.8636, -18.6251) ccw
  line L23 (-36.246, -16.5772) -> (-23.6374, -29.1331)
  arc A32 (-23.5625, -33.2372) -> (-23.6374, -29.1331) centre (-25.7596, -31.2246) ccw
  line L24 (-23.5625, -33.2372) -> (-55.4143, -68.0759)
  line L25 (5, -97.464) -> (5, -58.6595)
  arc A33 (7, -56.6595) -> (5, -58.6595) centre (7, -58.6595) ccw
  line L26 (7, -56.6595) -> (10.473, -56.6595)
  arc A34 (14.3032, -58.4456) -> (10.473, -56.6595) centre (10.473, -61.6595) ccw
  line L27 (14.3032, -58.4456) -> (34.3305, -82.3132)
  arc A35 (35.4243, -86.3954) -> (34.3305, -82.3132) centre (30.5003, -85.5271) ccw
  line L28 (35.4243, -86.3954) -> (32.7648, -101.4781)
  arc A36 (26.9725, -105.5339) -> (32.7648, -101.4781) centre (27.8408, -100.6098) ccw
  line L29 (26.9725, -105.5339) -> (9.1318, -102.3881)
  arc A37 (5, -97.464) -> (9.1318, -102.3881) centre (10, -97.464) ccw
  arc A38 (-40.9054, 16.7074) -> (-37.3489, 15.6517) centre (-38.8619, 17.0732) ccw
  line L30 (-40.9054, 16.7074) -> (-46.7322, 29.5993)
  arc A39 (-44.339, 36.0244) -> (-46.7322, 29.5993) centre (-42.0339, 31.5075) ccw
  arc A40 (-44.339, 36.0244) -> (-34.6129, 45.4956) centre (-56.2565, 57.9923) ccw
  arc A41 (-28.1234, 47.5076) -> (-34.6129, 45.4956) centre (-30.28, 42.9921) ccw
  line L31 (-28.1234, 47.5076) -> (-14.9942, 41.2515)
  arc A42 (-14.46, 38.0146) -> (-14.9942, 41.2515) centre (-15.8549, 39.4469) ccw
  line L32 (-14.46, 38.0146) -> (-37.3489, 15.6517)
  line L33 (70.4711, -73.2) -> (50.5773, -27.2494)
  arc A43 (51.0282, 29.3922) -> (50.5773, -27.2494) centre (114.8154, 0.5617) ccw
  line L34 (51.0282, 29.3922) -> (70.7852, 73.1043)
  arc A44 (70.7852, 73.1043) -> (60.1979, 89.9288) centre (75, 87.5) ccw
  arc A45 (35.9657, 79.8952) -> (60.1979, 89.9288) centre (-0.31, 201.7835) ccw
  arc A46 (-60.2098, 89.9999) -> (-70.7852, 73.1043) centre (-75, 87.5) ccw
  line L35 (-70.7852, 73.1043) -> (-51.0282, 29.3922)
  arc A47 (-50.5773, -27.2494) -> (-51.0282, 29.3922) centre (-114.8154, 0.5617) ccw
  line L36 (-50.5773, -27.2494) -> (-70.4711, -73.2)
  arc A48 (-70.4711, -73.2) -> (-73.7447, -102.4474) centre (-75, -87.5) ccw
  arc A49 (-46.7294, -108.889) -> (-73.7447, -102.4474) centre (-70.0264, -146.7235) ccw
  arc A50 (72.6915, -102.3213) -> (44.7852, -108.3244) centre (66.5604, -141.6847) ccw
  arc A51 (72.6915, -102.3213) -> (70.4711, -73.2) centre (75, -87.5) ccw
  arc A52 (-10.473, -56.6595) -> (-14.3032, -58.4456) centre (-10.473, -61.6595) ccw
  line L37 (-10.473, -56.6595) -> (-7, -56.6595)
  arc A53 (-5, -58.6595) -> (-7, -56.6595) centre (-7, -58.6595) ccw
  line L38 (-5, -58.6595) -> (-5, -97.464)
  arc A54 (-9.1318, -102.3881) -> (-5, -97.464) centre (-10, -97.464) ccw
  line L39 (-9.1318, -102.3881) -> (-26.9725, -105.5339)
  arc A55 (-32.7648, -101.4781) -> (-26.9725, -105.5339) centre (-27.8408, -100.6098) ccw
  line L40 (-32.7648, -101.4781) -> (-35.4243, -86.3954)
  arc A56 (-34.3305, -82.3132) -> (-35.4243, -86.3954) centre (-30.5003, -85.5271) ccw
  line L41 (-34.3305, -82.3132) -> (-14.3032, -58.4456)
  circle A57 centre (-40.65, 60) radius 2.15
  line L42 (47.15, 42.4858) -> (47.15, 67.561)
  arc A58 (49.4611, 71.7764) -> (47.15, 67.561) centre (52.15, 67.561) ccw
  line L43 (49.4611, 71.7764) -> (57.5607, 76.943)
  arc A59 (64.8173, 70.6939) -> (57.5607, 76.943) centre (60.2496, 72.7276) ccw
  line L44 (64.8173, 70.6939) -> (51.1653, 40.0309)
  arc A60 (49.5538, 39.7214) -> (51.1653, 40.0309) centre (50.2517, 40.4376) ccw
  line L45 (49.5538, 39.7214) -> (47.4521, 41.7697)
  arc A61 (47.15, 42.4858) -> (47.4521, 41.7697) centre (48.15, 42.4858) ccw
  circle A62 centre (40.65, 60) radius 2.15
  circle A63 centre (-40.65, 50) radius 2.15
  arc A64 (-57.5607, 76.943) -> (-64.8173, 70.6939) centre (-60.2496, 72.7276) ccw
  line L46 (-57.5607, 76.943) -> (-49.4611, 71.7764)
  arc A65 (-47.15, 67.561) -> (-49.4611, 71.7764) centre (-52.15, 67.561) ccw
  line L47 (-47.15, 67.561) -> (-47.15, 42.4858)
  arc A66 (-47.4521, 41.7697) -> (-47.15, 42.4858) centre (-48.15, 42.4858) ccw
  line L48 (-47.4521, 41.7697) -> (-49.5538, 39.7214)
  arc A67 (-51.1653, 40.0309) -> (-49.5538, 39.7214) centre (-50.2517, 40.4376) ccw
  line L49 (-51.1653, 40.0309) -> (-64.8173, 70.6939)
  circle A68 centre (40.65, 50) radius 2.15
  circle A69 centre (72.5, -79.6021) radius 1.5
  circle A70 centre (75, -87.5) radius 3
  circle A71 centre (-67, -87.4995) radius 1.5
  circle A72 centre (-74.9998, 79.5) radius 1.5
  circle A73 centre (67, 87.5) radius 1.5
  circle A74 centre (75, 87.5) radius 3
  circle A75 centre (75, 95.5) radius 1.5
  circle A76 centre (-83, 87.4998) radius 1.5
  circle A77 centre (-75, -87.5) radius 3
  circle A78 centre (80.5, -87.6021) radius 1.5
  circle A79 centre (64.5, -87.6021) radius 1.5
  circle A80 centre (-75.0005, -79.5) radius 1.5
  circle A81 centre (-74.9995, -95.5) radius 1.5
  circle A82 centre (-75, 87.5) radius 3
  circle A83 centre (75, 79.5) radius 1.5
  circle A84 centre (83, 87.5) radius 1.5
  circle A85 centre (-67, 87.5002) radius 1.5
  circle A86 centre (-75.0002, 95.5) radius 1.5
  circle A87 centre (-83, -87.5005) radius 1.5
  circle A88 centre (72.5, -95.6021) radius 1.5
  line L50 (75, 87.5) -> (96.2501, 66.2499) construction
  line L51 (75, 87.5) -> (104.2477, 87.5) construction
  line L52 (75, 87.5) -> (96.1586, 108.6586) construction
  line L53 (75, 87.5) -> (53.9343, 108.5657) construction
  circle A89 centre (85.6066, 76.8934) radius 6
  circle A90 centre (85.6066, 98.1066) radius 6
  circle A91 centre (64.3934, 98.1066) radius 6
  line L54 (-75, 87.5) -> (-58.7399, 103.7601) construction
  line L55 (-75, 87.5) -> (-51.2004, 87.5) construction
  line L56 (-75, 87.5) -> (-93.067, 105.567) construction
  line L57 (-75, 87.5) -> (-45.1095, 87.5) construction
  line L58 (-75, 87.5) -> (-91.323, 71.177) construction
  line L59 (75, -87.5) -> (90.3587, -102.8587) construction
  line L60 (75, -87.5) -> (92.7735, -69.7265) construction
  line L61 (-75, -87.5) -> (-99.4191, -111.9191) construction
  line L62 (-75, -87.5) -> (-36.2706, -87.5) construction
  line L63 (-75, -87.5) -> (-99.9358, -62.5642) construction
  circle A92 centre (-64.3934, 98.1066) radius 6
  circle A93 centre (-85.6066, 98.1066) radius 6
  circle A94 centre (-85.6066, 76.8934) radius 6
  circle A95 centre (85.6066, -76.8934) radius 6
  circle A96 centre (85.6066, -98.1066) radius 6
  line L64 (0, 0) -> (0, -47) construction
  circle A97 centre (-85.6066, -76.8934) radius 6
  circle A98 centre (-85.6066, -98.1066) radius 6
  line L65 (8.1464, -6.7322) -> (2.1213, -0.7071)
  arc A99 (2.1213, 0.7071) -> (2.1213, -0.7071) centre (2.8284, 0) ccw
  line L66 (2.1213, 0.7071) -> (8.1464, 6.7322)
  arc A100 (9, 6.3787) -> (8.1464, 6.7322) centre (8.5, 6.3787) ccw
  line L67 (9, 6.3787) -> (9, -6.3787)
  arc A101 (8.1464, -6.7322) -> (9, -6.3787) centre (8.5, -6.3787) ccw
  arc A102 (-6.7322, -8.1464) -> (-6.3787, -9) centre (-6.3787, -8.5) ccw
  line L68 (-6.7322, -8.1464) -> (-0.7071, -2.1213)
  arc A103 (0.7071, -2.1213) -> (-0.7071, -2.1213) centre (0, -2.8284) ccw
  line L69 (0.7071, -2.1213) -> (6.7322, -8.1464)
  arc A104 (6.3787, -9) -> (6.7322, -8.1464) centre (6.3787, -8.5) ccw
  line L70 (6.3787, -9) -> (-6.3787, -9)
  arc A105 (-8.1464, 6.7322) -> (-9, 6.3787) centre (-8.5, 6.3787) ccw
  line L71 (-8.1464, 6.7322) -> (-2.1213, 0.7071)
  arc A106 (-2.1213, -0.7071) -> (-2.1213, 0.7071) centre (-2.8284, 0) ccw
  line L72 (-2.1213, -0.7071) -> (-8.1464, -6.7322)
  arc A107 (-9, -6.3787) -> (-8.1464, -6.7322) centre (-8.5, -6.3787) ccw
  line L73 (-9, -6.3787) -> (-9, 6.3787)
  arc A108 (6.7322, 8.1464) -> (6.3787, 9) centre (6.3787, 8.5) ccw
  line L74 (6.7322, 8.1464) -> (0.7071, 2.1213)
  arc A109 (-0.7071, 2.1213) -> (0.7071, 2.1213) centre (0, 2.8284) ccw
  line L75 (-0.7071, 2.1213) -> (-6.7322, 8.1464)
  arc A110 (-6.3787, 9) -> (-6.7322, 8.1464) centre (-6.3787, 8.5) ccw
  line L76 (-6.3787, 9) -> (6.3787, 9)
  line L77 (35.9657, 79.8952) -> (2.1827, 93.0889)
  arc A111 (2.1827, 93.0889) -> (-2.1423, 93.1045) centre (0, 87.5) ccw
  line L78 (0, 81.5) -> (15.6612, 75.3836)
  line L79 (-16.4256, 75.2214) -> (0, 81.5)
  line L80 (-2.1423, 93.1045) -> (-36.9275, 79.8081)
  arc A112 (-60.2098, 89.9999) -> (-36.7745, 80.3179) centre (-0.31, 201.7835) ccw
  circle A113 centre (0, 87.5) radius 2.15
  arc A114 (26.2105, 50.915) -> (27.5676, 55.0697) centre (24.9353, 53.6305) ccw
  line L81 (26.2105, 50.915) -> (10.6059, 43.5872)
  arc A115 (9.3307, 43.3027) -> (10.6059, 43.5872) centre (9.3307, 46.3027) ccw
  line L82 (9.3307, 43.3027) -> (-9.3218, 43.3027)
  arc A116 (-10.6123, 43.5944) -> (-9.3218, 43.3027) centre (-9.3218, 46.3027) ccw
  line L83 (-10.6123, 43.5944) -> (-26.8632, 51.3381)
  arc A117 (-28.1945, 55.5044) -> (-26.8632, 51.3381) centre (-25.5727, 54.0463) ccw
  line L84 (-28.1945, 55.5044) -> (-17.9762, 73.8773)
  arc A118 (-16.4256, 75.2214) -> (-17.9762, 73.8773) centre (-15.3544, 72.4192) ccw
  arc A119 (17.2021, 74.0283) -> (15.6612, 75.3836) centre (14.5698, 72.5892) ccw
  line L85 (17.2021, 74.0283) -> (27.5676, 55.0697)
  arc A120 (-46.7294, -108.889) -> (-25.7561, -114.8285) centre (-25.7561, -74.8285) ccw
  line L86 (-25.7561, -114.8285) -> (22.9214, -114.8285)
  arc A121 (22.9214, -114.8285) -> (44.7852, -108.3244) centre (22.9214, -74.8285) ccw
  circle A122 centre (10, 10) radius 3
  circle A123 centre (-10, -10) radius 3
  circle A124 centre (10, -10) radius 3
  circle A125 centre (-10, 10) radius 3
  point P0 (0.156, 201.9423)
  point P1 (72.5, -87.6021)
  point P2 (72.5, 87.3979)
  point P3 (-72.5, -87.6021)
  point P4 (-72.5, 87.3979)
  point P5 (0.156, 201.9423)
  point P6 (72.5, -87.6021)
  point P7 (72.5, 87.3979)
  point P8 (-72.5, -87.6021)
  point P9 (-72.5, 87.3979)
  point P10 (0.156, 201.9423)
  point P11 (72.5, -87.6021)
  point P12 (72.5, 87.3979)
  point P13 (-72.5, -87.6021)
  point P14 (-72.5, 87.3979)
  point P15 (0.2929, 201.9885)
  point P16 (72.5, -87.6021)
  point P17 (72.5, 87.3979)
  point P18 (-72.5, -87.6021)
  point P19 (-72.5, 87.3979)
  point P20 (0.2929, 201.9885)
  point P21 (72.5, -87.6021)
  point P22 (72.5, 87.3979)
  point P23 (-72.5, -87.6021)
  point P24 (-72.5, 87.3979)
  point P25 (0.2929, 201.9885)
  point P26 (72.5, -87.6021)
  point P27 (0.2929, 201.9885)
  point P28 (72.5, -87.6021)
  point P29 (2.2046, 200.8918)
  point P30 (72.5, -87.6021)
  point P31 (2.2046, 200.8918)
  point P32 (72.5, -87.6021)
  dimension "d120" = 45
  dimension "d121" = 12
  dimension "d122" = 12
  dimension "d123" = 12
  dimension "d126" = 45
  dimension "d127" = 135
  dimension "d128" = 135
  dimension "d129" = 12
  dimension "d130" = 12
  dimension "d131" = 12
  dimension "d134" = 12
  dimension "d135" = 12
  constraint horizontal L51
  constraint coincident A44.centre A74.centre
  constraint perpendicular L50 L52
  constraint perpendicular L52 L53
  constraint coincident L50 A89.centre
  constraint coincident A44 A89.centre
  constraint coincident L52 A90.centre
  constraint coincident A44 A90.centre
  constraint coincident A44 A91.centre
  constraint coincident L53 A91.centre
  constraint horizontal L55
  constraint coincident A46.centre A82.centre
  constraint horizontal L57
  constraint perpendicular L56 L58
  constraint coincident A51.centre A70.centre
  constraint perpendicular L58 L59
  constraint perpendicular L59 L60
  constraint horizontal L62
  constraint coincident A48.centre A77.centre
  constraint perpendicular L61 L63
  constraint coincident L54 A92.centre
  constraint coincident A46 A92.centre
  constraint coincident L56 A93.centre
  constraint coincident A46 A93.centre
  constraint coincident L58 A94.centre
  constraint coincident A46 A94.centre
  constraint coincident A51 A95.centre
  constraint coincident L60 A95.centre
  constraint coincident L59 A96.centre
  constraint coincident A51 A96.centre
  constraint coincident L64.start origin
  constraint perpendicular L1 L64
  constraint symmetric A95 L64 A97
  constraint symmetric A96 L64 A98
  measures "d120" angle of L50 L51
  measures "d121" diameter of A89
  measures "d122" diameter of A90
  measures "d123" diameter of A91
  measures "d126" angle of L54 L55
  measures "d127" angle of L56 L57
  measures "d128" angle of L61 L62
  measures "d129" diameter of A92
  measures "d130" diameter of A93
  measures "d131" diameter of A94
  measures "d134" diameter of A95
  measures "d135" diameter of A96
extrude "Extrusão6" cut sketch "Esboço6" against normal blind 10 contours A44 A89 | A44 A90 | A44 A91 picked at (84.9701, 79.0831) picked at (83.4169, 97.4701) picked at (66.5772, 97.4609)
extrude "Extrusão7" cut sketch "Esboço6" against normal blind 50 contours A44 A89 | A44 A90 | A44 A91 | A46 A92 | A46 A93 | A46 A94 picked at (84.9701, 79.0831) picked at (83.4169, 97.4701) picked at (66.5772, 97.4609) picked at (-65.0299, 95.9169) picked at (-83.4228, 97.4609) picked at (-83.4228, 77.5391)
extrude "Extrusão8" cut sketch "Esboço6" against normal blind 22 contours A48 A97 | A48 A98 | A51 A96 | A51 A95 picked at (-83.4228, -77.5391) picked at (-83.4228, -97.4609) picked at (84.9701, -95.9169) picked at (84.9701, -79.0831)
fillet "Arredondamento1" radius 50 6 edges at (-70.4711, 73.2, 0) (-60.1979, -89.9288, 0) (-70.7852, -73.1043, 0) (60.2098, -89.9999, 0) (70.7852, -73.1043, 0) (70.4711, 73.2, 0)
fillet "Arredondamento2" radius 3 20 edges at (-80.6012, 73.585, 0) (-88.915, 81.8988, 0) (-88.915, 93.1012, 0) (-80.6012, 101.415, 0) (-80.6012, -73.585, 0) (-88.915, -81.8988, 0) (-80.6012, -101.415, 0) (-88.915, -93.1012, 0) (-69.3988, -101.415, 0) (-61.085, -93.1012, 0) (61.085, -93.1012, 0) (69.3988, -101.415, 0) (88.915, -93.1012, 0) (80.6012, -101.415, 0) (80.6012, -73.585, 0) (88.915, -81.8988, 0) (80.6012, 73.585, 0) (88.915, 81.8988, 0) (80.6012, 101.415, 0) (88.915, 93.1012, 0)